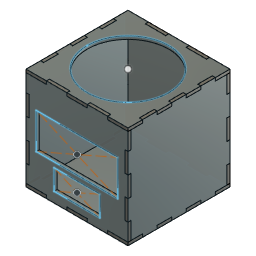
BaseholderFinalProject (Autodesk Fusion 360 design; units mm, degrees)
Autodesk Fusion 360 part; units mm, degrees
sketch "Sketch1" plane through (0, 0, 0) normal (0, 1, 0) x (1, 0, 0) in component "base"
  line L0 (0, 0) -> (100, 0)
  line L1 (100, 0) -> (100, 100)
  line L2 (100, 100) -> (0, 100)
  line L3 (0, 100) -> (0, 0)
  dimension "d1" = 100
  dimension "d2" = 100
  constraint horizontal L0
  constraint vertical L1
  constraint horizontal L2
  constraint vertical L3
  constraint coincident L0.start L3.end
  measures "d1" distance of L0.start L0.end
  measures "d2" distance of L0.start L2.end
extrude "Extrude1" add sketch "Sketch1" along normal blind 3 makes body 1 in component "base"
sketch "Sketch1 (2)" plane through (0, 0, 0) normal (0, 0, 1) x (1, 0, 0) in component "side1"
  line L0 (0, 0) -> (100, 0)
  line L1 (100, 0) -> (100, 3)
  line L2 (100, 3) -> (0, 3)
  line L3 (0, 3) -> (0, 0)
  line L4 (0, 0) -> (100, 0)
  line L5 (100, 0) -> (100, 100)
  line L6 (100, 100) -> (0, 100)
  line L7 (0, 100) -> (0, 0)
  line L8 (0, 3) -> (100, 3)
  line L9 (20, 3) -> (20, 0)
  line L10 (40, 3) -> (40, 0)
  line L11 (60, 3) -> (60, 0)
  line L12 (80, 3) -> (80, 0)
  dimension "d9" = 100
  dimension "d10" = 100
  dimension "d51" = 3
  dimension "d52" = 20
  dimension "d55" = 20
  dimension "d56" = 0
  constraint horizontal L4
  constraint vertical L5
  constraint horizontal L6
  constraint vertical L7
  constraint coincident L0.start L3.end
  constraint coincident L7 L2.end
  constraint coincident L5 L1.end
  constraint perpendicular L5 L8
  constraint coincident L2 L9.start
  constraint coincident L4 L9.end
  constraint perpendicular L4 L9
  measures "d9" distance of L0.start L0.end
  measures "d10" distance of L0.start L6.end
  measures "d51" distance of L4 L8
  measures "d52" distance of L7 L9
extrude "Extrude1'" add sketch "Sketch1 (2)" against normal blind 3 separate body contours L0 L2 L4 L8 L9 L10 | L2 L5 L6 L7 L8 | L0 L2 L4 L8 L11 L12 makes body 2 in component "side1"
sketch "Sketch1 (3)" plane through (100, 0, 0) normal (1, 0, 0) x (0, 0, -1) in component "front"
  line L0 (0, 0) -> (100, 0)
  line L1 (100, 0) -> (100, 3)
  line L2 (100, 3) -> (0, 3)
  line L3 (0, 3) -> (0, 0)
  line L4 (0, 0) -> (100, 0)
  line L5 (100, 0) -> (100, 100)
  line L6 (100, 100) -> (0, 100)
  line L7 (0, 100) -> (0, 0)
  line L8 (3, 100) -> (3, 0)
  line L9 (97, 100) -> (97, 0)
  line L10 (100, 3) -> (0, 3)
  line L11 (0, 20) -> (3, 20)
  line L12 (0, 40) -> (3, 40)
  line L13 (0, 60) -> (3, 60)
  line L14 (0, 80) -> (3, 80)
  line L15 (97, 20) -> (100, 20)
  line L16 (14.2857, 3) -> (14.2857, 0)
  line L17 (28.5714, 3) -> (28.5714, 0)
  line L18 (42.8571, 3) -> (42.8571, 0)
  line L19 (57.1429, 3) -> (57.1429, 0)
  line L20 (71.4286, 3) -> (71.4286, 0)
  line L21 (85.7143, 3) -> (85.7143, 0)
  line L22 (100, 3) -> (100, 0)
  line L23 (114.2857, 3) -> (114.2857, 0)
  line L24 (97, 40) -> (100, 40)
  line L25 (97, 60) -> (100, 60)
  line L26 (97, 80) -> (100, 80)
  dimension "d13" = 100
  dimension "d14" = 100
  dimension "d25" = 3
  dimension "d26" = 3
  dimension "d27" = 3
  dimension "d28" = 20
  dimension "d31" = -20
  dimension "d32" = 0
  dimension "d33" = 20
  dimension "d38" = 14.2857
  dimension "d41" = 14.2857
  dimension "d42" = 0
  dimension "d49" = 20
  dimension "d50" = 0
  constraint horizontal L4
  constraint vertical L5
  constraint horizontal L6
  constraint vertical L7
  constraint coincident L0.start L3.end
  constraint coincident L6 L8.start
  constraint coincident L4 L8.end
  constraint perpendicular L4 L8
  constraint coincident L6 L9.start
  constraint coincident L0 L9.end
  constraint perpendicular L0 L9
  constraint coincident L5 L1.end
  constraint coincident L7 L2.end
  constraint perpendicular L7 L10
  constraint coincident L7 L11.start
  constraint coincident L8 L11.end
  constraint perpendicular L8 L11
  constraint coincident L9 L15.start
  constraint coincident L5 L15.end
  constraint perpendicular L5 L15
  constraint coincident L10 L16.start
  constraint coincident L4 L16.end
  constraint perpendicular L4 L16
  measures "d13" distance of L0.start L0.end
  measures "d14" distance of L0.start L6.end
  measures "d25" distance of L7 L8
  measures "d26" distance of L5 L9
  measures "d27" distance of L4 L10
  measures "d28" distance of L4 L11
  measures "d33" distance of L4 L15
  measures "d38" distance of L7 L16
extrude "Extrude1''" add sketch "Sketch1 (3)" against normal blind 3 separate body contours L0 L2 L4 L10 L16 L17 | L2 L6 L8 L9 L10 | L7 L8 L11 L12 | L0 L2 L4 L10 L18 L19 | L7 L8 L13 L14 | L0 L2 L4 L10 L20 L21 | L5 L9 L25 L26 | L5 L9 L15 L24 makes body 3 in component "front"
pattern_linear "R-Pattern1" count 2 spacing 97 along (0, 0, -1) of bodies 2 makes body 4 in component "side1"
pattern_linear "R-Pattern1'" count 2 spacing 97 along (-1, 0, 0) of bodies 3 makes body 5 in component "front"
combine "Combine1" operation cut target body 1 tool bodies 4 3 2 5 keep tools in component "base"
combine "Combine1'" operation cut target body 2 tool bodies 5 3 keep tools in component "side1"
combine "Combine2" operation cut target body 4 tool bodies 5 3 keep tools in component "side1"
pattern_linear "R-Pattern2" count 2 spacing 97 along (0, 1, 0) of bodies 1 makes body 6 in component "base"
combine "Combine3" operation cut target body 2 tool bodies 6 keep tools in component "side1"
combine "Combine4" operation cut target body 4 tool bodies 6 keep tools in component "side1"
combine "Combine1''" operation cut target body 5 tool bodies 6 keep tools in component "front"
combine "Combine2'" operation cut target body 3 tool bodies 6 keep tools in component "front"
sketch "bottom" plane through (0, 0, 0) normal (0, -1, 0) x (1, 0, 0)
  line L0 (0, -14.2857) -> (3, -14.2857)
  line L1 (3, -14.2857) -> (3, -28.5714)
  line L2 (3, -28.5714) -> (0, -28.5714)
  line L3 (0, -28.5714) -> (0, -42.8571)
  line L4 (0, -42.8571) -> (3, -42.8571)
  line L5 (3, -42.8571) -> (3, -57.1429)
  line L6 (3, -57.1429) -> (0, -57.1429)
  line L7 (0, -57.1429) -> (0, -71.4286)
  line L8 (0, -71.4286) -> (3, -71.4286)
  line L9 (3, -71.4286) -> (3, -85.7143)
  line L10 (3, -85.7143) -> (0, -85.7143)
  line L11 (0, -85.7143) -> (0, -100)
  line L12 (0, -100) -> (20, -100)
  line L13 (20, -100) -> (20, -97)
  line L14 (20, -97) -> (40, -97)
  line L15 (40, -97) -> (40, -100)
  line L16 (40, -100) -> (60, -100)
  line L17 (60, -100) -> (60, -97)
  line L18 (60, -97) -> (80, -97)
  line L19 (80, -97) -> (80, -100)
  line L20 (80, -100) -> (100, -100)
  line L21 (100, -100) -> (100, -85.7143)
  line L22 (100, -85.7143) -> (97, -85.7143)
  line L23 (97, -85.7143) -> (97, -71.4286)
  line L24 (97, -71.4286) -> (100, -71.4286)
  line L25 (100, -71.4286) -> (100, -57.1429)
  line L26 (100, -57.1429) -> (97, -57.1429)
  line L27 (97, -57.1429) -> (97, -42.8571)
  line L28 (97, -42.8571) -> (100, -42.8571)
  line L29 (100, -42.8571) -> (100, -28.5714)
  line L30 (100, -28.5714) -> (97, -28.5714)
  line L31 (97, -28.5714) -> (97, -14.2857)
  line L32 (97, -14.2857) -> (100, -14.2857)
  line L33 (100, -14.2857) -> (100, 0)
  line L34 (100, 0) -> (80, 0)
  line L35 (80, 0) -> (80, -3)
  line L36 (80, -3) -> (60, -3)
  line L37 (60, -3) -> (60, 0)
  line L38 (60, 0) -> (40, 0)
  line L39 (40, 0) -> (40, -3)
  line L40 (40, -3) -> (20, -3)
  line L41 (20, -3) -> (20, 0)
  line L42 (20, 0) -> (0, 0)
  line L43 (0, 0) -> (0, -14.2857)
sketch "front" plane through (0, 0, 0) normal (0, 0, 1) x (1, 0, 0)
  line L0 (100, 97) -> (80, 97)
  line L1 (80, 97) -> (80, 100)
  line L2 (80, 100) -> (60, 100)
  line L3 (60, 100) -> (60, 97)
  line L4 (60, 97) -> (40, 97)
  line L5 (40, 97) -> (40, 100)
  line L6 (40, 100) -> (20, 100)
  line L7 (20, 100) -> (20, 97)
  line L8 (20, 97) -> (0, 97)
  line L9 (0, 97) -> (0, 80)
  line L10 (0, 80) -> (3, 80)
  line L11 (3, 80) -> (3, 60)
  line L12 (3, 60) -> (0, 60)
  line L13 (0, 60) -> (0, 40)
  line L14 (0, 40) -> (3, 40)
  line L15 (3, 40) -> (3, 20)
  line L16 (3, 20) -> (0, 20)
  line L17 (0, 20) -> (0, 3)
  line L18 (0, 3) -> (20, 3)
  line L19 (20, 3) -> (20, 0)
  line L20 (20, 0) -> (40, 0)
  line L21 (40, 0) -> (40, 3)
  line L22 (40, 3) -> (60, 3)
  line L23 (60, 3) -> (60, 0)
  line L24 (60, 0) -> (80, 0)
  line L25 (80, 0) -> (80, 3)
  line L26 (80, 3) -> (100, 3)
  line L27 (100, 3) -> (100, 20)
  line L28 (100, 20) -> (97, 20)
  line L29 (97, 20) -> (97, 40)
  line L30 (97, 40) -> (100, 40)
  line L31 (100, 40) -> (100, 60)
  line L32 (100, 60) -> (97, 60)
  line L33 (97, 60) -> (97, 80)
  line L34 (97, 80) -> (100, 80)
  line L35 (100, 80) -> (100, 97)
  line L36 (72.5, 30) -> (27.5, 30)
  line L37 (27.5, 30) -> (27.5, 10)
  line L38 (27.5, 10) -> (72.5, 10)
  line L39 (72.5, 10) -> (72.5, 30)
  line L40 (72.5, 30) -> (27.5, 10) construction
  line L41 (27.5, 30) -> (72.5, 10) construction
  line L42 (90, 35) -> (10, 35)
  line L43 (10, 35) -> (10, 70)
  line L44 (10, 70) -> (90, 70)
  line L45 (90, 70) -> (90, 35)
  line L46 (90, 35) -> (10, 70) construction
  line L47 (10, 35) -> (90, 70) construction
  point P0 (50, 20)
  point P1 (50, 52.5)
  dimension "d74" = 45
  dimension "d75" = 20
  dimension "d76" = 80
  dimension "d77" = 35
  dimension "d78" = 5
  constraint horizontal L36
  constraint perpendicular L36 L37
  constraint parallel L36 L38
  constraint parallel L37 L39
  constraint coincident L40 P0
  constraint coincident L41 P0
  constraint horizontal L42
  constraint perpendicular L42 L43
  constraint parallel L42 L44
  constraint parallel L43 L45
  constraint coincident L46 P1
  constraint coincident L47 P1
  measures "d74" distance of L37.end L38.end
  measures "d75" distance of L36.end L37.end
  measures "d76" distance of L43.end L44.end
  measures "d77" distance of L42.end L43.end
  measures "d78" distance of L36 L42
extrude "Extrude2" cut sketch "front" against normal blind 3 contours L36 L37 L38 L39 | L42 L43 L44 L45 bodies 2 in component "side1"
sketch "top" plane through (0, 100, 0) normal (0, 1, 0) x (-1, 0, 0)
  line L0 (0, -14.2857) -> (0, 0)
  line L1 (0, 0) -> (-20, 0)
  line L2 (-20, 0) -> (-20, -3)
  line L3 (-20, -3) -> (-40, -3)
  line L4 (-40, -3) -> (-40, 0)
  line L5 (-40, 0) -> (-60, 0)
  line L6 (-60, 0) -> (-60, -3)
  line L7 (-60, -3) -> (-80, -3)
  line L8 (-80, -3) -> (-80, 0)
  line L9 (-80, 0) -> (-100, 0)
  line L10 (-100, 0) -> (-100, -14.2857)
  line L11 (-100, -14.2857) -> (-97, -14.2857)
  line L12 (-97, -14.2857) -> (-97, -28.5714)
  line L13 (-97, -28.5714) -> (-100, -28.5714)
  line L14 (-100, -28.5714) -> (-100, -42.8571)
  line L15 (-100, -42.8571) -> (-97, -42.8571)
  line L16 (-97, -42.8571) -> (-97, -57.1429)
  line L17 (-97, -57.1429) -> (-100, -57.1429)
  line L18 (-100, -57.1429) -> (-100, -71.4286)
  line L19 (-100, -71.4286) -> (-97, -71.4286)
  line L20 (-97, -71.4286) -> (-97, -85.7143)
  line L21 (-97, -85.7143) -> (-100, -85.7143)
  line L22 (-100, -85.7143) -> (-100, -100)
  line L23 (-100, -100) -> (-80, -100)
  line L24 (-80, -100) -> (-80, -97)
  line L25 (-80, -97) -> (-60, -97)
  line L26 (-60, -97) -> (-60, -100)
  line L27 (-60, -100) -> (-40, -100)
  line L28 (-40, -100) -> (-40, -97)
  line L29 (-40, -97) -> (-20, -97)
  line L30 (-20, -97) -> (-20, -100)
  line L31 (-20, -100) -> (0, -100)
  line L32 (0, -100) -> (0, -85.7143)
  line L33 (0, -85.7143) -> (-3, -85.7143)
  line L34 (-3, -85.7143) -> (-3, -71.4286)
  line L35 (-3, -71.4286) -> (0, -71.4286)
  line L36 (0, -71.4286) -> (0, -57.1429)
  line L37 (0, -57.1429) -> (-3, -57.1429)
  line L38 (-3, -57.1429) -> (-3, -42.8571)
  line L39 (-3, -42.8571) -> (0, -42.8571)
  line L40 (0, -42.8571) -> (0, -28.5714)
  line L41 (0, -28.5714) -> (-3, -28.5714)
  line L42 (-3, -28.5714) -> (-3, -14.2857)
  line L43 (-3, -14.2857) -> (0, -14.2857)
  circle A0 centre (-50, -50) radius 40
  dimension "d81" = 80
  measures "d81" diameter of A0
extrude "Extrude2'" cut sketch "top" against normal blind 3 contours A0 bodies 6 in component "base"
sketch "side1" plane through (100, 0, 0) normal (1, 0, 0) x (0, 0, -1)
  line L0 (14.2857, 97) -> (3, 97)
  line L1 (3, 97) -> (3, 80)
  line L2 (3, 80) -> (0, 80)
  line L3 (0, 80) -> (0, 60)
  line L4 (0, 60) -> (3, 60)
  line L5 (3, 60) -> (3, 40)
  line L6 (3, 40) -> (0, 40)
  line L7 (0, 40) -> (0, 20)
  line L8 (0, 20) -> (3, 20)
  line L9 (3, 20) -> (3, 3)
  line L10 (3, 3) -> (14.2857, 3)
  line L11 (14.2857, 3) -> (14.2857, 0)
  line L12 (14.2857, 0) -> (28.5714, 0)
  line L13 (28.5714, 0) -> (28.5714, 3)
  line L14 (28.5714, 3) -> (42.8571, 3)
  line L15 (42.8571, 3) -> (42.8571, 0)
  line L16 (42.8571, 0) -> (57.1429, 0)
  line L17 (57.1429, 0) -> (57.1429, 3)
  line L18 (57.1429, 3) -> (71.4286, 3)
  line L19 (71.4286, 3) -> (71.4286, 0)
  line L20 (71.4286, 0) -> (85.7143, 0)
  line L21 (85.7143, 0) -> (85.7143, 3)
  line L22 (85.7143, 3) -> (97, 3)
  line L23 (97, 3) -> (97, 20)
  line L24 (97, 20) -> (100, 20)
  line L25 (100, 20) -> (100, 40)
  line L26 (100, 40) -> (97, 40)
  line L27 (97, 40) -> (97, 60)
  line L28 (97, 60) -> (100, 60)
  line L29 (100, 60) -> (100, 80)
  line L30 (100, 80) -> (97, 80)
  line L31 (97, 80) -> (97, 97)
  line L32 (97, 97) -> (85.7143, 97)
  line L33 (85.7143, 97) -> (85.7143, 100)
  line L34 (85.7143, 100) -> (71.4286, 100)
  line L35 (71.4286, 100) -> (71.4286, 97)
  line L36 (71.4286, 97) -> (57.1429, 97)
  line L37 (57.1429, 97) -> (57.1429, 100)
  line L38 (57.1429, 100) -> (42.8571, 100)
  line L39 (42.8571, 100) -> (42.8571, 97)
  line L40 (42.8571, 97) -> (28.5714, 97)
  line L41 (28.5714, 97) -> (28.5714, 100)
  line L42 (28.5714, 100) -> (14.2857, 100)
  line L43 (14.2857, 100) -> (14.2857, 97)
sketch "side2" plane through (0, 0, 0) normal (-1, 0, 0) x (0, 0, 1)
  line L0 (-85.7143, 97) -> (-97, 97)
  line L1 (-97, 97) -> (-97, 80)
  line L2 (-97, 80) -> (-100, 80)
  line L3 (-100, 80) -> (-100, 60)
  line L4 (-100, 60) -> (-97, 60)
  line L5 (-97, 60) -> (-97, 40)
  line L6 (-97, 40) -> (-100, 40)
  line L7 (-100, 40) -> (-100, 20)
  line L8 (-100, 20) -> (-97, 20)
  line L9 (-97, 20) -> (-97, 3)
  line L10 (-97, 3) -> (-85.7143, 3)
  line L11 (-85.7143, 3) -> (-85.7143, 0)
  line L12 (-85.7143, 0) -> (-71.4286, 0)
  line L13 (-71.4286, 0) -> (-71.4286, 3)
  line L14 (-71.4286, 3) -> (-57.1429, 3)
  line L15 (-57.1429, 3) -> (-57.1429, 0)
  line L16 (-57.1429, 0) -> (-42.8571, 0)
  line L17 (-42.8571, 0) -> (-42.8571, 3)
  line L18 (-42.8571, 3) -> (-28.5714, 3)
  line L19 (-28.5714, 3) -> (-28.5714, 0)
  line L20 (-28.5714, 0) -> (-14.2857, 0)
  line L21 (-14.2857, 0) -> (-14.2857, 3)
  line L22 (-14.2857, 3) -> (-3, 3)
  line L23 (-3, 3) -> (-3, 20)
  line L24 (-3, 20) -> (0, 20)
  line L25 (0, 20) -> (0, 40)
  line L26 (0, 40) -> (-3, 40)
  line L27 (-3, 40) -> (-3, 60)
  line L28 (-3, 60) -> (0, 60)
  line L29 (0, 60) -> (0, 80)
  line L30 (0, 80) -> (-3, 80)
  line L31 (-3, 80) -> (-3, 97)
  line L32 (-3, 97) -> (-14.2857, 97)
  line L33 (-14.2857, 97) -> (-14.2857, 100)
  line L34 (-14.2857, 100) -> (-28.5714, 100)
  line L35 (-28.5714, 100) -> (-28.5714, 97)
  line L36 (-28.5714, 97) -> (-42.8571, 97)
  line L37 (-42.8571, 97) -> (-42.8571, 100)
  line L38 (-42.8571, 100) -> (-57.1429, 100)
  line L39 (-57.1429, 100) -> (-57.1429, 97)
  line L40 (-57.1429, 97) -> (-71.4286, 97)
  line L41 (-71.4286, 97) -> (-71.4286, 100)
  line L42 (-71.4286, 100) -> (-85.7143, 100)
  line L43 (-85.7143, 100) -> (-85.7143, 97)
sketch "behind" plane through (0, 0, -100) normal (0, 0, -1) x (-1, 0, 0)
  line L0 (0, 97) -> (-20, 97)
  line L1 (-20, 97) -> (-20, 100)
  line L2 (-20, 100) -> (-40, 100)
  line L3 (-40, 100) -> (-40, 97)
  line L4 (-40, 97) -> (-60, 97)
  line L5 (-60, 97) -> (-60, 100)
  line L6 (-60, 100) -> (-80, 100)
  line L7 (-80, 100) -> (-80, 97)
  line L8 (-80, 97) -> (-100, 97)
  line L9 (-100, 97) -> (-100, 80)
  line L10 (-100, 80) -> (-97, 80)
  line L11 (-97, 80) -> (-97, 60)
  line L12 (-97, 60) -> (-100, 60)
  line L13 (-100, 60) -> (-100, 40)
  line L14 (-100, 40) -> (-97, 40)
  line L15 (-97, 40) -> (-97, 20)
  line L16 (-97, 20) -> (-100, 20)
  line L17 (-100, 20) -> (-100, 3)
  line L18 (-100, 3) -> (-80, 3)
  line L19 (-80, 3) -> (-80, 0)
  line L20 (-80, 0) -> (-60, 0)
  line L21 (-60, 0) -> (-60, 3)
  line L22 (-60, 3) -> (-40, 3)
  line L23 (-40, 3) -> (-40, 0)
  line L24 (-40, 0) -> (-20, 0)
  line L25 (-20, 0) -> (-20, 3)
  line L26 (-20, 3) -> (0, 3)
  line L27 (0, 3) -> (0, 20)
  line L28 (0, 20) -> (-3, 20)
  line L29 (-3, 20) -> (-3, 40)
  line L30 (-3, 40) -> (0, 40)
  line L31 (0, 40) -> (0, 60)
  line L32 (0, 60) -> (-3, 60)
  line L33 (-3, 60) -> (-3, 80)
  line L34 (-3, 80) -> (0, 80)
  line L35 (0, 80) -> (0, 97)
  circle A0 centre (-30, 20) radius 10
  dimension "d84" = 20
  measures "d84" diameter of A0
extrude "Extrude3" cut sketch "behind" against normal blind 3 contours A0 bodies 4 in component "side1"
component "base" placed x (1, 0, 0) y (0, 1, 0) z (0, 0, 1) at (0, 0, 0)
component "side1" placed x (1, 0, 0) y (0, 1, 0) z (0, 0, 1) at (0, 0, 0)
component "front" placed x (1, 0, 0) y (0, 1, 0) z (0, 0, 1) at (0, 0, 0)
equation "d1 = width"
equation "d2 = width"
equation "d3 = thickness"
equation "width = 100 mm"
equation "depth = 50 mm"
equation "height = 100 mm"
equation "thickness = 3 mm"
equation "d9 = width"
equation "d10 = height"
equation "d11 = -thickness"
equation "d13 = width"
equation "d14 = height"
equation "d15 = -thickness"
equation "d19 = width - thickness"
equation "d23 = -( width - thickness )"
equation "d25 = thickness"
equation "d26 = thickness"
equation "d27 = thickness"
equation "d28 = height / 5"
equation "d31 = -( height / 5 )"
equation "d33 = height / 5"
equation "d38 = width / 7"
equation "d41 = width / 7"
equation "d49 = height / 5"
equation "d51 = thickness"
equation "d52 = width / 5"
equation "d55 = width / 5"
equation "d63 = height - thickness"
equation "d79 = -thickness"
equation "d82 = -thickness"
equation "d85 = -thickness"
